Autodesk Fusion 360 part; units mm, degrees
(part 6 of 10)
sketch "Sketch33" plane through (0, 0, 9) normal (0, 0, 1) x (-1, 0, 0)
  line L0 (-20, 20.68) -> (-20, 19.68)
  line L1 (-20, 19.68) -> (-21, 19.68)
  line L2 (-21, 19.68) -> (-21, 20.68)
  line L3 (-21, 20.68) -> (-20, 20.68)
  line L4 (-23, 20.68) -> (-23, 19.68)
  line L5 (-23, 19.68) -> (-24, 19.68)
  line L6 (-24, 19.68) -> (-24, 20.68)
  line L7 (-24, 20.68) -> (-23, 20.68)
  line L8 (-20, 18.05) -> (-20, 17.05)
  line L9 (-20, 17.05) -> (-21, 17.05)
  line L10 (-21, 17.05) -> (-21, 18.05)
  line L11 (-21, 18.05) -> (-20, 18.05)
  line L12 (-23, 18.05) -> (-23, 17.05)
  line L13 (-23, 17.05) -> (-24, 17.05)
  line L14 (-24, 17.05) -> (-24, 18.05)
  line L15 (-24, 18.05) -> (-23, 18.05)
  line L16 (-20, 15.42) -> (-20, 14.42)
  line L17 (-20, 14.42) -> (-21, 14.42)
  line L18 (-21, 14.42) -> (-21, 15.42)
  line L19 (-21, 15.42) -> (-20, 15.42)
  line L20 (-23, 15.42) -> (-23, 14.42)
  line L21 (-23, 14.42) -> (-24, 14.42)
  line L22 (-24, 14.42) -> (-24, 15.42)
  line L23 (-24, 15.42) -> (-23, 15.42)
  line L24 (-20, 12.79) -> (-20, 11.79)
  line L25 (-20, 11.79) -> (-21, 11.79)
  line L26 (-21, 11.79) -> (-21, 12.79)
  line L27 (-21, 12.79) -> (-20, 12.79)
  line L28 (-23, 12.79) -> (-23, 11.79)
  line L29 (-23, 11.79) -> (-24, 11.79)
  line L30 (-24, 11.79) -> (-24, 12.79)
  line L31 (-24, 12.79) -> (-23, 12.79)
  line L32 (-20, 10.16) -> (-20, 9.16)
  line L33 (-20, 9.16) -> (-21, 9.16)
  line L34 (-21, 9.16) -> (-21, 10.16)
  line L35 (-21, 10.16) -> (-20, 10.16)
  line L36 (-23, 10.16) -> (-23, 9.16)
  line L37 (-23, 9.16) -> (-24, 9.16)
  line L38 (-24, 9.16) -> (-24, 10.16)
  line L39 (-24, 10.16) -> (-23, 10.16)
  line L40 (-19.998, 5.46) -> (-19.998, 4.46)
  line L41 (-19.998, 4.46) -> (-20.998, 4.46)
  line L42 (-20.998, 4.46) -> (-20.998, 5.46)
  line L43 (-20.998, 5.46) -> (-19.998, 5.46)
  line L44 (-22.998, 5.46) -> (-22.998, 4.46)
  line L45 (-22.998, 4.46) -> (-23.998, 4.46)
  line L46 (-23.998, 4.46) -> (-23.998, 5.46)
  line L47 (-23.998, 5.46) -> (-22.998, 5.46)
  line L48 (-19.998, 2.83) -> (-19.998, 1.83)
  line L49 (-19.998, 1.83) -> (-20.998, 1.83)
  line L50 (-20.998, 1.83) -> (-20.998, 2.83)
  line L51 (-20.998, 2.83) -> (-19.998, 2.83)
  line L52 (-22.998, 2.83) -> (-22.998, 1.83)
  line L53 (-22.998, 1.83) -> (-23.998, 1.83)
  line L54 (-23.998, 1.83) -> (-23.998, 2.83)
  line L55 (-23.998, 2.83) -> (-22.998, 2.83)
  line L56 (-19.998, 0.2) -> (-19.998, -0.8)
  line L57 (-19.998, -0.8) -> (-20.998, -0.8)
  line L58 (-20.998, -0.8) -> (-20.998, 0.2)
  line L59 (-20.998, 0.2) -> (-19.998, 0.2)
  line L60 (-22.998, 0.2) -> (-22.998, -0.8)
  line L61 (-22.998, -0.8) -> (-23.998, -0.8)
  line L62 (-23.998, -0.8) -> (-23.998, 0.2)
  line L63 (-23.998, 0.2) -> (-22.998, 0.2)
  line L64 (-19.998, -2.43) -> (-19.998, -3.43)
  line L65 (-19.998, -3.43) -> (-20.998, -3.43)
  line L66 (-20.998, -3.43) -> (-20.998, -2.43)
  line L67 (-20.998, -2.43) -> (-19.998, -2.43)
  line L68 (-22.998, -2.43) -> (-22.998, -3.43)
  line L69 (-22.998, -3.43) -> (-23.998, -3.43)
  line L70 (-23.998, -3.43) -> (-23.998, -2.43)
  line L71 (-23.998, -2.43) -> (-22.998, -2.43)
  line L72 (-19.998, -5.06) -> (-19.998, -6.06)
  line L73 (-19.998, -6.06) -> (-20.998, -6.06)
  line L74 (-20.998, -6.06) -> (-20.998, -5.06)
  line L75 (-20.998, -5.06) -> (-19.998, -5.06)
  line L76 (-22.998, -5.06) -> (-22.998, -6.06)
  line L77 (-22.998, -6.06) -> (-23.998, -6.06)
  line L78 (-23.998, -6.06) -> (-23.998, -5.06)
  line L79 (-23.998, -5.06) -> (-22.998, -5.06)
  line L80 (-20, -9.76) -> (-20, -10.76)
  line L81 (-20, -10.76) -> (-21, -10.76)
  line L82 (-21, -10.76) -> (-21, -9.76)
  line L83 (-21, -9.76) -> (-20, -9.76)
  line L84 (-23, -9.76) -> (-23, -10.76)
  line L85 (-23, -10.76) -> (-24, -10.76)
  line L86 (-24, -10.76) -> (-24, -9.76)
  line L87 (-24, -9.76) -> (-23, -9.76)
  line L88 (-20, -12.39) -> (-20, -13.39)
  line L89 (-20, -13.39) -> (-21, -13.39)
  line L90 (-21, -13.39) -> (-21, -12.39)
  line L91 (-21, -12.39) -> (-20, -12.39)
  line L92 (-23, -12.39) -> (-23, -13.39)
  line L93 (-23, -13.39) -> (-24, -13.39)
  line L94 (-24, -13.39) -> (-24, -12.39)
  line L95 (-24, -12.39) -> (-23, -12.39)
  line L96 (-20, -15.02) -> (-20, -16.02)
  line L97 (-20, -16.02) -> (-21, -16.02)
  line L98 (-21, -16.02) -> (-21, -15.02)
  line L99 (-21, -15.02) -> (-20, -15.02)
  line L100 (-23, -15.02) -> (-23, -16.02)
  line L101 (-23, -16.02) -> (-24, -16.02)
  line L102 (-24, -16.02) -> (-24, -15.02)
  line L103 (-24, -15.02) -> (-23, -15.02)
  line L104 (-20, -17.65) -> (-20, -18.65)
  line L105 (-20, -18.65) -> (-21, -18.65)
  line L106 (-21, -18.65) -> (-21, -17.65)
  line L107 (-21, -17.65) -> (-20, -17.65)
  line L108 (-23, -17.65) -> (-23, -18.65)
  line L109 (-23, -18.65) -> (-24, -18.65)
  line L110 (-24, -18.65) -> (-24, -17.65)
  line L111 (-24, -17.65) -> (-23, -17.65)
  line L112 (-20, -20.28) -> (-20, -21.28)
  line L113 (-20, -21.28) -> (-21, -21.28)
  line L114 (-21, -21.28) -> (-21, -20.28)
  line L115 (-21, -20.28) -> (-20, -20.28)
  line L116 (-23, -20.28) -> (-23, -21.28)
  line L117 (-23, -21.28) -> (-24, -21.28)
  line L118 (-24, -21.28) -> (-24, -20.28)
  line L119 (-24, -20.28) -> (-23, -20.28)
  line L120 (-20, -24.98) -> (-20, -25.98)
  line L121 (-20, -25.98) -> (-21, -25.98)
  line L122 (-21, -25.98) -> (-21, -24.98)
  line L123 (-21, -24.98) -> (-20, -24.98)
  line L124 (-23, -24.98) -> (-23, -25.98)
  line L125 (-23, -25.98) -> (-24, -25.98)
  line L126 (-24, -25.98) -> (-24, -24.98)
  line L127 (-24, -24.98) -> (-23, -24.98)
  line L128 (-20, -27.61) -> (-20, -28.61)
  line L129 (-20, -28.61) -> (-21, -28.61)
  line L130 (-21, -28.61) -> (-21, -27.61)
  line L131 (-21, -27.61) -> (-20, -27.61)
  line L132 (-23, -27.61) -> (-23, -28.61)
  line L133 (-23, -28.61) -> (-24, -28.61)
  line L134 (-24, -28.61) -> (-24, -27.61)
  line L135 (-24, -27.61) -> (-23, -27.61)
  line L136 (-20, -30.24) -> (-20, -31.24)
  line L137 (-20, -31.24) -> (-21, -31.24)
  line L138 (-21, -31.24) -> (-21, -30.24)
  line L139 (-21, -30.24) -> (-20, -30.24)
  line L140 (-23, -30.24) -> (-23, -31.24)
  line L141 (-23, -31.24) -> (-24, -31.24)
  line L142 (-24, -31.24) -> (-24, -30.24)
  line L143 (-24, -30.24) -> (-23, -30.24)
  line L144 (-20, -32.87) -> (-20, -33.87)
  line L145 (-20, -33.87) -> (-21, -33.87)
  line L146 (-21, -33.87) -> (-21, -32.87)
  line L147 (-21, -32.87) -> (-20, -32.87)
  line L148 (-23, -32.87) -> (-23, -33.87)
  line L149 (-23, -33.87) -> (-24, -33.87)
  line L150 (-24, -33.87) -> (-24, -32.87)
  line L151 (-24, -32.87) -> (-23, -32.87)
  line L152 (-20, -35.5) -> (-20, -36.5)
  line L153 (-20, -36.5) -> (-21, -36.5)
  line L154 (-21, -36.5) -> (-21, -35.5)
  line L155 (-21, -35.5) -> (-20, -35.5)
  line L156 (-23, -35.5) -> (-23, -36.5)
  line L157 (-23, -36.5) -> (-24, -36.5)
  line L158 (-24, -36.5) -> (-24, -35.5)
  line L159 (-24, -35.5) -> (-23, -35.5)
  line L160 (-13.7, 38.77) -> (-13.7, 37.77)
  line L161 (-13.7, 37.77) -> (-14.7, 37.77)
  line L162 (-14.7, 37.77) -> (-14.7, 38.77)
  line L163 (-14.7, 38.77) -> (-13.7, 38.77)
  line L164 (-13.7, 36.14) -> (-13.7, 35.14)
  line L165 (-13.7, 35.14) -> (-14.7, 35.14)
  line L166 (-14.7, 35.14) -> (-14.7, 36.14)
  line L167 (-14.7, 36.14) -> (-13.7, 36.14)
  line L168 (-13.7, 33.51) -> (-13.7, 32.51)
  line L169 (-13.7, 32.51) -> (-14.7, 32.51)
  line L170 (-14.7, 32.51) -> (-14.7, 33.51)
  line L171 (-14.7, 33.51) -> (-13.7, 33.51)
  line L172 (-13.7, 30.88) -> (-13.7, 29.88)
  line L173 (-13.7, 29.88) -> (-14.7, 29.88)
  line L174 (-14.7, 29.88) -> (-14.7, 30.88)
  line L175 (-14.7, 30.88) -> (-13.7, 30.88)
  line L176 (-13.7, 28.25) -> (-13.7, 27.25)
  line L177 (-13.7, 27.25) -> (-14.7, 27.25)
  line L178 (-14.7, 27.25) -> (-14.7, 28.25)
  line L179 (-14.7, 28.25) -> (-13.7, 28.25)
  line L180 (-13.7, 25.62) -> (-13.7, 24.62)
  line L181 (-13.7, 24.62) -> (-14.7, 24.62)
  line L182 (-14.7, 24.62) -> (-14.7, 25.62)
  line L183 (-14.7, 25.62) -> (-13.7, 25.62)
  line L184 (-13.7, 22.99) -> (-13.7, 21.99)
  line L185 (-13.7, 21.99) -> (-14.7, 21.99)
  line L186 (-14.7, 21.99) -> (-14.7, 22.99)
  line L187 (-14.7, 22.99) -> (-13.7, 22.99)
  line L188 (-13.7, 20.36) -> (-13.7, 19.36)
  line L189 (-13.7, 19.36) -> (-14.7, 19.36)
  line L190 (-14.7, 19.36) -> (-14.7, 20.36)
  line L191 (-14.7, 20.36) -> (-13.7, 20.36)
  line L192 (-13.7, 17.73) -> (-13.7, 16.73)
  line L193 (-13.7, 16.73) -> (-14.7, 16.73)
  line L194 (-14.7, 16.73) -> (-14.7, 17.73)
  line L195 (-14.7, 17.73) -> (-13.7, 17.73)
  line L196 (-13.7, 15.1) -> (-13.7, 14.1)
  line L197 (-13.7, 14.1) -> (-14.7, 14.1)
  line L198 (-14.7, 14.1) -> (-14.7, 15.1)
  line L199 (-14.7, 15.1) -> (-13.7, 15.1)
  line L200 (-13.7, 12.47) -> (-13.7, 11.47)
  line L201 (-13.7, 11.47) -> (-14.7, 11.47)
  line L202 (-14.7, 11.47) -> (-14.7, 12.47)
  line L203 (-14.7, 12.47) -> (-13.7, 12.47)
  line L204 (-13.7, 9.84) -> (-13.7, 8.84)
  line L205 (-13.7, 8.84) -> (-14.7, 8.84)
  line L206 (-14.7, 8.84) -> (-14.7, 9.84)
  line L207 (-14.7, 9.84) -> (-13.7, 9.84)
  line L208 (-13.7, 7.21) -> (-13.7, 6.21)
  line L209 (-13.7, 6.21) -> (-14.7, 6.21)
  line L210 (-14.7, 6.21) -> (-14.7, 7.21)
  line L211 (-14.7, 7.21) -> (-13.7, 7.21)
  line L212 (-13.7, 4.58) -> (-13.7, 3.58)
  line L213 (-13.7, 3.58) -> (-14.7, 3.58)
  line L214 (-14.7, 3.58) -> (-14.7, 4.58)
  line L215 (-14.7, 4.58) -> (-13.7, 4.58)
  line L216 (-13.7, 1.95) -> (-13.7, 0.95)
  line L217 (-13.7, 0.95) -> (-14.7, 0.95)
  line L218 (-14.7, 0.95) -> (-14.7, 1.95)
  line L219 (-14.7, 1.95) -> (-13.7, 1.95)
  line L220 (-13.7, -0.68) -> (-13.7, -1.68)
  line L221 (-13.7, -1.68) -> (-14.7, -1.68)
  line L222 (-14.7, -1.68) -> (-14.7, -0.68)
  line L223 (-14.7, -0.68) -> (-13.7, -0.68)
  line L224 (-13.7, -3.31) -> (-13.7, -4.31)
  line L225 (-13.7, -4.31) -> (-14.7, -4.31)
  line L226 (-14.7, -4.31) -> (-14.7, -3.31)
  line L227 (-14.7, -3.31) -> (-13.7, -3.31)
  line L228 (-13.7, -5.94) -> (-13.7, -6.94)
  line L229 (-13.7, -6.94) -> (-14.7, -6.94)
  line L230 (-14.7, -6.94) -> (-14.7, -5.94)
  line L231 (-14.7, -5.94) -> (-13.7, -5.94)
  line L232 (-13.7, -8.57) -> (-13.7, -9.57)
  line L233 (-13.7, -9.57) -> (-14.7, -9.57)
  line L234 (-14.7, -9.57) -> (-14.7, -8.57)
  line L235 (-14.7, -8.57) -> (-13.7, -8.57)
  line L236 (-13.7, -11.2) -> (-13.7, -12.2)
  line L237 (-13.7, -12.2) -> (-14.7, -12.2)
  line L238 (-14.7, -12.2) -> (-14.7, -11.2)
  line L239 (-14.7, -11.2) -> (-13.7, -11.2)
  line L240 (-13.7, -13.83) -> (-13.7, -14.83)
  line L241 (-13.7, -14.83) -> (-14.7, -14.83)
  line L242 (-14.7, -14.83) -> (-14.7, -13.83)
  line L243 (-14.7, -13.83) -> (-13.7, -13.83)
  line L244 (-13.7, -16.46) -> (-13.7, -17.46)
  line L245 (-13.7, -17.46) -> (-14.7, -17.46)
  line L246 (-14.7, -17.46) -> (-14.7, -16.46)
  line L247 (-14.7, -16.46) -> (-13.7, -16.46)
  line L248 (-13.7, -19.09) -> (-13.7, -20.09)
  line L249 (-13.7, -20.09) -> (-14.7, -20.09)
  line L250 (-14.7, -20.09) -> (-14.7, -19.09)
  line L251 (-14.7, -19.09) -> (-13.7, -19.09)
  line L252 (-13.7, -21.72) -> (-13.7, -22.72)
  line L253 (-13.7, -22.72) -> (-14.7, -22.72)
  line L254 (-14.7, -22.72) -> (-14.7, -21.72)
  line L255 (-14.7, -21.72) -> (-13.7, -21.72)
  line L256 (-13.7, -24.35) -> (-13.7, -25.35)
  line L257 (-13.7, -25.35) -> (-14.7, -25.35)
  line L258 (-14.7, -25.35) -> (-14.7, -24.35)
  line L259 (-14.7, -24.35) -> (-13.7, -24.35)
  line L260 (-13.7, -26.98) -> (-13.7, -27.98)
  line L261 (-13.7, -27.98) -> (-14.7, -27.98)
  line L262 (-14.7, -27.98) -> (-14.7, -26.98)
  line L263 (-14.7, -26.98) -> (-13.7, -26.98)
  line L264 (-13.7, -29.61) -> (-13.7, -30.61)
  line L265 (-13.7, -30.61) -> (-14.7, -30.61)
  line L266 (-14.7, -30.61) -> (-14.7, -29.61)
  line L267 (-14.7, -29.61) -> (-13.7, -29.61)
  line L268 (-13.7, -32.24) -> (-13.7, -33.24)
  line L269 (-13.7, -33.24) -> (-14.7, -33.24)
  line L270 (-14.7, -33.24) -> (-14.7, -32.24)
  line L271 (-14.7, -32.24) -> (-13.7, -32.24)
  line L272 (-13.7, -34.87) -> (-13.7, -35.87)
  line L273 (-13.7, -35.87) -> (-14.7, -35.87)
  line L274 (-14.7, -35.87) -> (-14.7, -34.87)
  line L275 (-14.7, -34.87) -> (-13.7, -34.87)
  line L276 (-13.7, -37.5) -> (-13.7, -38.5)
  line L277 (-13.7, -38.5) -> (-14.7, -38.5)
  line L278 (-14.7, -38.5) -> (-14.7, -37.5)
  line L279 (-14.7, -37.5) -> (-13.7, -37.5)
  line L280 (-10.9, 38.77) -> (-10.9, 37.77)
  line L281 (-10.9, 37.77) -> (-11.9, 37.77)
  line L282 (-11.9, 37.77) -> (-11.9, 38.77)
  line L283 (-11.9, 38.77) -> (-10.9, 38.77)
  line L284 (-10.9, 36.14) -> (-10.9, 35.14)
  line L285 (-10.9, 35.14) -> (-11.9, 35.14)
  line L286 (-11.9, 35.14) -> (-11.9, 36.14)
  line L287 (-11.9, 36.14) -> (-10.9, 36.14)
  line L288 (-10.9, 33.51) -> (-10.9, 32.51)
  line L289 (-10.9, 32.51) -> (-11.9, 32.51)
  line L290 (-11.9, 32.51) -> (-11.9, 33.51)
  line L291 (-11.9, 33.51) -> (-10.9, 33.51)
  line L292 (-10.9, 30.88) -> (-10.9, 29.88)
  line L293 (-10.9, 29.88) -> (-11.9, 29.88)
  line L294 (-11.9, 29.88) -> (-11.9, 30.88)
  line L295 (-11.9, 30.88) -> (-10.9, 30.88)
  line L296 (-10.9, 28.25) -> (-10.9, 27.25)
  line L297 (-10.9, 27.25) -> (-11.9, 27.25)
  line L298 (-11.9, 27.25) -> (-11.9, 28.25)
  line L299 (-11.9, 28.25) -> (-10.9, 28.25)
  line L300 (-10.9, 25.62) -> (-10.9, 24.62)
  line L301 (-10.9, 24.62) -> (-11.9, 24.62)
  line L302 (-11.9, 24.62) -> (-11.9, 25.62)
  line L303 (-11.9, 25.62) -> (-10.9, 25.62)
  line L304 (-10.9, 22.99) -> (-10.9, 21.99)
  line L305 (-10.9, 21.99) -> (-11.9, 21.99)
  line L306 (-11.9, 21.99) -> (-11.9, 22.99)
  line L307 (-11.9, 22.99) -> (-10.9, 22.99)
  line L308 (-10.9, 20.36) -> (-10.9, 19.36)
  line L309 (-10.9, 19.36) -> (-11.9, 19.36)
  line L310 (-11.9, 19.36) -> (-11.9, 20.36)
  line L311 (-11.9, 20.36) -> (-10.9, 20.36)
  line L312 (-10.9, 17.73) -> (-10.9, 16.73)
  line L313 (-10.9, 16.73) -> (-11.9, 16.73)
  line L314 (-11.9, 16.73) -> (-11.9, 17.73)
  line L315 (-11.9, 17.73) -> (-10.9, 17.73)
  line L316 (-10.9, 15.1) -> (-10.9, 14.1)
  line L317 (-10.9, 14.1) -> (-11.9, 14.1)
  line L318 (-11.9, 14.1) -> (-11.9, 15.1)
  line L319 (-11.9, 15.1) -> (-10.9, 15.1)
  line L320 (-10.9, 12.47) -> (-10.9, 11.47)
  line L321 (-10.9, 11.47) -> (-11.9, 11.47)
  line L322 (-11.9, 11.47) -> (-11.9, 12.47)
  line L323 (-11.9, 12.47) -> (-10.9, 12.47)
  line L324 (-10.9, 9.84) -> (-10.9, 8.84)
  line L325 (-10.9, 8.84) -> (-11.9, 8.84)
  line L326 (-11.9, 8.84) -> (-11.9, 9.84)
  line L327 (-11.9, 9.84) -> (-10.9, 9.84)
  line L328 (-10.9, 7.21) -> (-10.9, 6.21)
  line L329 (-10.9, 6.21) -> (-11.9, 6.21)
  line L330 (-11.9, 6.21) -> (-11.9, 7.21)
  line L331 (-11.9, 7.21) -> (-10.9, 7.21)
  line L332 (-10.9, 4.58) -> (-10.9, 3.58)
  line L333 (-10.9, 3.58) -> (-11.9, 3.58)
  line L334 (-11.9, 3.58) -> (-11.9, 4.58)
  line L335 (-11.9, 4.58) -> (-10.9, 4.58)
  line L336 (-10.9, 1.95) -> (-10.9, 0.95)
  line L337 (-10.9, 0.95) -> (-11.9, 0.95)
  line L338 (-11.9, 0.95) -> (-11.9, 1.95)
  line L339 (-11.9, 1.95) -> (-10.9, 1.95)
  line L340 (-10.9, -0.68) -> (-10.9, -1.68)
  line L341 (-10.9, -1.68) -> (-11.9, -1.68)
  line L342 (-11.9, -1.68) -> (-11.9, -0.68)
  line L343 (-11.9, -0.68) -> (-10.9, -0.68)
  line L344 (-10.9, -3.31) -> (-10.9, -4.31)
  line L345 (-10.9, -4.31) -> (-11.9, -4.31)
  line L346 (-11.9, -4.31) -> (-11.9, -3.31)
  line L347 (-11.9, -3.31) -> (-10.9, -3.31)
  line L348 (-10.9, -5.94) -> (-10.9, -6.94)
  line L349 (-10.9, -6.94) -> (-11.9, -6.94)
  line L350 (-11.9, -6.94) -> (-11.9, -5.94)
  line L351 (-11.9, -5.94) -> (-10.9, -5.94)
  line L352 (-10.9, -8.57) -> (-10.9, -9.57)
  line L353 (-10.9, -9.57) -> (-11.9, -9.57)
  line L354 (-11.9, -9.57) -> (-11.9, -8.57)
  line L355 (-11.9, -8.57) -> (-10.9, -8.57)
  line L356 (-10.9, -11.2) -> (-10.9, -12.2)
  line L357 (-10.9, -12.2) -> (-11.9, -12.2)
  line L358 (-11.9, -12.2) -> (-11.9, -11.2)
  line L359 (-11.9, -11.2) -> (-10.9, -11.2)
  line L360 (-10.9, -13.83) -> (-10.9, -14.83)
  line L361 (-10.9, -14.83) -> (-11.9, -14.83)
  line L362 (-11.9, -14.83) -> (-11.9, -13.83)
  line L363 (-11.9, -13.83) -> (-10.9, -13.83)
  line L364 (-10.9, -16.46) -> (-10.9, -17.46)
  line L365 (-10.9, -17.46) -> (-11.9, -17.46)
  line L366 (-11.9, -17.46) -> (-11.9, -16.46)
  line L367 (-11.9, -16.46) -> (-10.9, -16.46)
  line L368 (-10.9, -19.09) -> (-10.9, -20.09)
  line L369 (-10.9, -20.09) -> (-11.9, -20.09)
  line L370 (-11.9, -20.09) -> (-11.9, -19.09)
  line L371 (-11.9, -19.09) -> (-10.9, -19.09)
  line L372 (-10.9, -21.72) -> (-10.9, -22.72)
  line L373 (-10.9, -22.72) -> (-11.9, -22.72)
  line L374 (-11.9, -22.72) -> (-11.9, -21.72)
  line L375 (-11.9, -21.72) -> (-10.9, -21.72)
  line L376 (-10.9, -24.35) -> (-10.9, -25.35)
  line L377 (-10.9, -25.35) -> (-11.9, -25.35)
  line L378 (-11.9, -25.35) -> (-11.9, -24.35)
  line L379 (-11.9, -24.35) -> (-10.9, -24.35)
  line L380 (-10.9, -26.98) -> (-10.9, -27.98)
  line L381 (-10.9, -27.98) -> (-11.9, -27.98)
  line L382 (-11.9, -27.98) -> (-11.9, -26.98)
  line L383 (-11.9, -26.98) -> (-10.9, -26.98)
  line L384 (-10.9, -29.61) -> (-10.9, -30.61)
  line L385 (-10.9, -30.61) -> (-11.9, -30.61)
  line L386 (-11.9, -30.61) -> (-11.9, -29.61)
  line L387 (-11.9, -29.61) -> (-10.9, -29.61)
  line L388 (-10.9, -32.24) -> (-10.9, -33.24)
  line L389 (-10.9, -33.24) -> (-11.9, -33.24)
  line L390 (-11.9, -33.24) -> (-11.9, -32.24)
  line L391 (-11.9, -32.24) -> (-10.9, -32.24)
  line L392 (-10.9, -34.87) -> (-10.9, -35.87)
  line L393 (-10.9, -35.87) -> (-11.9, -35.87)
  line L394 (-11.9, -35.87) -> (-11.9, -34.87)
  line L395 (-11.9, -34.87) -> (-10.9, -34.87)
  line L396 (-10.9, -37.5) -> (-10.9, -38.5)
  line L397 (-10.9, -38.5) -> (-11.9, -38.5)
  line L398 (-11.9, -38.5) -> (-11.9, -37.5)
  line L399 (-11.9, -37.5) -> (-10.9, -37.5)
  line L400 (-8.1, 38.77) -> (-8.1, 37.77)
  line L401 (-8.1, 37.77) -> (-9.1, 37.77)
  line L402 (-9.1, 37.77) -> (-9.1, 38.77)
  line L403 (-9.1, 38.77) -> (-8.1, 38.77)
  line L404 (-8.1, 36.14) -> (-8.1, 35.14)
  line L405 (-8.1, 35.14) -> (-9.1, 35.14)
  line L406 (-9.1, 35.14) -> (-9.1, 36.14)
  line L407 (-9.1, 36.14) -> (-8.1, 36.14)
  line L408 (-8.1, 33.51) -> (-8.1, 32.51)
  line L409 (-8.1, 32.51) -> (-9.1, 32.51)
  line L410 (-9.1, 32.51) -> (-9.1, 33.51)
  line L411 (-9.1, 33.51) -> (-8.1, 33.51)
  line L412 (-8.1, 30.88) -> (-8.1, 29.88)
  line L413 (-8.1, 29.88) -> (-9.1, 29.88)
  line L414 (-9.1, 29.88) -> (-9.1, 30.88)
  line L415 (-9.1, 30.88) -> (-8.1, 30.88)
  line L416 (-8.1, 28.25) -> (-8.1, 27.25)
  line L417 (-8.1, 27.25) -> (-9.1, 27.25)
  line L418 (-9.1, 27.25) -> (-9.1, 28.25)
  line L419 (-9.1, 28.25) -> (-8.1, 28.25)
  line L420 (-8.1, 25.62) -> (-8.1, 24.62)
  line L421 (-8.1, 24.62) -> (-9.1, 24.62)
  line L422 (-9.1, 24.62) -> (-9.1, 25.62)
  line L423 (-9.1, 25.62) -> (-8.1, 25.62)
  line L424 (-8.1, 22.99) -> (-8.1, 21.99)
  line L425 (-8.1, 21.99) -> (-9.1, 21.99)
  line L426 (-9.1, 21.99) -> (-9.1, 22.99)
  line L427 (-9.1, 22.99) -> (-8.1, 22.99)
  line L428 (-8.1, 20.36) -> (-8.1, 19.36)
  line L429 (-8.1, 19.36) -> (-9.1, 19.36)
  line L430 (-9.1, 19.36) -> (-9.1, 20.36)
  line L431 (-9.1, 20.36) -> (-8.1, 20.36)
  line L432 (-8.1, 17.73) -> (-8.1, 16.73)
  line L433 (-8.1, 16.73) -> (-9.1, 16.73)
  line L434 (-9.1, 16.73) -> (-9.1, 17.73)
  line L435 (-9.1, 17.73) -> (-8.1, 17.73)
  line L436 (-8.1, 15.1) -> (-8.1, 14.1)
  line L437 (-8.1, 14.1) -> (-9.1, 14.1)
  line L438 (-9.1, 14.1) -> (-9.1, 15.1)
  line L439 (-9.1, 15.1) -> (-8.1, 15.1)
  line L440 (-8.1, 12.47) -> (-8.1, 11.47)
  line L441 (-8.1, 11.47) -> (-9.1, 11.47)
  line L442 (-9.1, 11.47) -> (-9.1, 12.47)
  line L443 (-9.1, 12.47) -> (-8.1, 12.47)
  line L444 (-8.1, 9.84) -> (-8.1, 8.84)
  line L445 (-8.1, 8.84) -> (-9.1, 8.84)
  line L446 (-9.1, 8.84) -> (-9.1, 9.84)
  line L447 (-9.1, 9.84) -> (-8.1, 9.84)
  line L448 (-8.1, 7.21) -> (-8.1, 6.21)
  line L449 (-8.1, 6.21) -> (-9.1, 6.21)
  line L450 (-9.1, 6.21) -> (-9.1, 7.21)
  line L451 (-9.1, 7.21) -> (-8.1, 7.21)
  line L452 (-8.1, 4.58) -> (-8.1, 3.58)
  line L453 (-8.1, 3.58) -> (-9.1, 3.58)
  line L454 (-9.1, 3.58) -> (-9.1, 4.58)
  line L455 (-9.1, 4.58) -> (-8.1, 4.58)
  line L456 (-8.1, 1.95) -> (-8.1, 0.95)
  line L457 (-8.1, 0.95) -> (-9.1, 0.95)
  line L458 (-9.1, 0.95) -> (-9.1, 1.95)
  line L459 (-9.1, 1.95) -> (-8.1, 1.95)
  line L460 (-8.1, -0.68) -> (-8.1, -1.68)
  line L461 (-8.1, -1.68) -> (-9.1, -1.68)
  line L462 (-9.1, -1.68) -> (-9.1, -0.68)
  line L463 (-9.1, -0.68) -> (-8.1, -0.68)
  line L464 (-8.1, -3.31) -> (-8.1, -4.31)
  line L465 (-8.1, -4.31) -> (-9.1, -4.31)
  line L466 (-9.1, -4.31) -> (-9.1, -3.31)
  line L467 (-9.1, -3.31) -> (-8.1, -3.31)
  line L468 (-8.1, -5.94) -> (-8.1, -6.94)
  line L469 (-8.1, -6.94) -> (-9.1, -6.94)
  line L470 (-9.1, -6.94) -> (-9.1, -5.94)
  line L471 (-9.1, -5.94) -> (-8.1, -5.94)
  line L472 (-8.1, -8.57) -> (-8.1, -9.57)
  line L473 (-8.1, -9.57) -> (-9.1, -9.57)
  line L474 (-9.1, -9.57) -> (-9.1, -8.57)
  line L475 (-9.1, -8.57) -> (-8.1, -8.57)
  line L476 (-8.1, -11.2) -> (-8.1, -12.2)
  line L477 (-8.1, -12.2) -> (-9.1, -12.2)
  line L478 (-9.1, -12.2) -> (-9.1, -11.2)
  line L479 (-9.1, -11.2) -> (-8.1, -11.2)
  line L480 (-8.1, -13.83) -> (-8.1, -14.83)
  line L481 (-8.1, -14.83) -> (-9.1, -14.83)
  line L482 (-9.1, -14.83) -> (-9.1, -13.83)
  line L483 (-9.1, -13.83) -> (-8.1, -13.83)
  line L484 (-8.1, -16.46) -> (-8.1, -17.46)
  line L485 (-8.1, -17.46) -> (-9.1, -17.46)
  line L486 (-9.1, -17.46) -> (-9.1, -16.46)
  line L487 (-9.1, -16.46) -> (-8.1, -16.46)
  line L488 (-8.1, -19.09) -> (-8.1, -20.09)
  line L489 (-8.1, -20.09) -> (-9.1, -20.09)
  line L490 (-9.1, -20.09) -> (-9.1, -19.09)
  line L491 (-9.1, -19.09) -> (-8.1, -19.09)
  line L492 (-8.1, -21.72) -> (-8.1, -22.72)
  line L493 (-8.1, -22.72) -> (-9.1, -22.72)
  line L494 (-9.1, -22.72) -> (-9.1, -21.72)
  line L495 (-9.1, -21.72) -> (-8.1, -21.72)
  line L496 (-8.1, -24.35) -> (-8.1, -25.35)
  line L497 (-8.1, -25.35) -> (-9.1, -25.35)
  line L498 (-9.1, -25.35) -> (-9.1, -24.35)
  line L499 (-9.1, -24.35) -> (-8.1, -24.35)
  line L500 (-8.1, -26.98) -> (-8.1, -27.98)
  line L501 (-8.1, -27.98) -> (-9.1, -27.98)
  line L502 (-9.1, -27.98) -> (-9.1, -26.98)
  line L503 (-9.1, -26.98) -> (-8.1, -26.98)
  line L504 (-8.1, -29.61) -> (-8.1, -30.61)
  line L505 (-8.1, -30.61) -> (-9.1, -30.61)
  line L506 (-9.1, -30.61) -> (-9.1, -29.61)
  line L507 (-9.1, -29.61) -> (-8.1, -29.61)
  line L508 (-8.1, -32.24) -> (-8.1, -33.24)
  line L509 (-8.1, -33.24) -> (-9.1, -33.24)
  line L510 (-9.1, -33.24) -> (-9.1, -32.24)
  line L511 (-9.1, -32.24) -> (-8.1, -32.24)
  line L512 (-8.1, -34.87) -> (-8.1, -35.87)
  line L513 (-8.1, -35.87) -> (-9.1, -35.87)
  line L514 (-9.1, -35.87) -> (-9.1, -34.87)
  line L515 (-9.1, -34.87) -> (-8.1, -34.87)
  line L516 (-8.1, -37.5) -> (-8.1, -38.5)
  line L517 (-8.1, -38.5) -> (-9.1, -38.5)
  line L518 (-9.1, -38.5) -> (-9.1, -37.5)
  line L519 (-9.1, -37.5) -> (-8.1, -37.5)
  line L520 (-5.3, 38.77) -> (-5.3, 37.77)
  line L521 (-5.3, 37.77) -> (-6.3, 37.77)
  line L522 (-6.3, 37.77) -> (-6.3, 38.77)
  line L523 (-6.3, 38.77) -> (-5.3, 38.77)
  line L524 (-5.3, 36.14) -> (-5.3, 35.14)
  line L525 (-5.3, 35.14) -> (-6.3, 35.14)
  line L526 (-6.3, 35.14) -> (-6.3, 36.14)
  line L527 (-6.3, 36.14) -> (-5.3, 36.14)
  line L528 (-5.3, 33.51) -> (-5.3, 32.51)
  line L529 (-5.3, 32.51) -> (-6.3, 32.51)
  line L530 (-6.3, 32.51) -> (-6.3, 33.51)
  line L531 (-6.3, 33.51) -> (-5.3, 33.51)
  line L532 (-5.3, 30.88) -> (-5.3, 29.88)
  line L533 (-5.3, 29.88) -> (-6.3, 29.88)
  line L534 (-6.3, 29.88) -> (-6.3, 30.88)
  line L535 (-6.3, 30.88) -> (-5.3, 30.88)
  line L536 (-5.3, 28.25) -> (-5.3, 27.25)
  line L537 (-5.3, 27.25) -> (-6.3, 27.25)
  line L538 (-6.3, 27.25) -> (-6.3, 28.25)
  line L539 (-6.3, 28.25) -> (-5.3, 28.25)
  line L540 (-5.3, 25.62) -> (-5.3, 24.62)
  line L541 (-5.3, 24.62) -> (-6.3, 24.62)
  line L542 (-6.3, 24.62) -> (-6.3, 25.62)
  line L543 (-6.3, 25.62) -> (-5.3, 25.62)
  line L544 (-5.3, 22.99) -> (-5.3, 21.99)
  line L545 (-5.3, 21.99) -> (-6.3, 21.99)
  line L546 (-6.3, 21.99) -> (-6.3, 22.99)
  line L547 (-6.3, 22.99) -> (-5.3, 22.99)
  line L548 (-5.3, 20.36) -> (-5.3, 19.36)
  line L549 (-5.3, 19.36) -> (-6.3, 19.36)
  line L550 (-6.3, 19.36) -> (-6.3, 20.36)
  line L551 (-6.3, 20.36) -> (-5.3, 20.36)
  line L552 (-5.3, 17.73) -> (-5.3, 16.73)
  line L553 (-5.3, 16.73) -> (-6.3, 16.73)
  line L554 (-6.3, 16.73) -> (-6.3, 17.73)
  line L555 (-6.3, 17.73) -> (-5.3, 17.73)
  line L556 (-5.3, 15.1) -> (-5.3, 14.1)
  line L557 (-5.3, 14.1) -> (-6.3, 14.1)
  line L558 (-6.3, 14.1) -> (-6.3, 15.1)
  line L559 (-6.3, 15.1) -> (-5.3, 15.1)
  line L560 (-5.3, 12.47) -> (-5.3, 11.47)
  line L561 (-5.3, 11.47) -> (-6.3, 11.47)
  line L562 (-6.3, 11.47) -> (-6.3, 12.47)
  line L563 (-6.3, 12.47) -> (-5.3, 12.47)
  line L564 (-5.3, 9.84) -> (-5.3, 8.84)
  line L565 (-5.3, 8.84) -> (-6.3, 8.84)
  line L566 (-6.3, 8.84) -> (-6.3, 9.84)
  line L567 (-6.3, 9.84) -> (-5.3, 9.84)
  line L568 (-5.3, 7.21) -> (-5.3, 6.21)
  line L569 (-5.3, 6.21) -> (-6.3, 6.21)
  line L570 (-6.3, 6.21) -> (-6.3, 7.21)
  line L571 (-6.3, 7.21) -> (-5.3, 7.21)
  line L572 (-5.3, 4.58) -> (-5.3, 3.58)
  line L573 (-5.3, 3.58) -> (-6.3, 3.58)
  line L574 (-6.3, 3.58) -> (-6.3, 4.58)
  line L575 (-6.3, 4.58) -> (-5.3, 4.58)
  line L576 (-5.3, 1.95) -> (-5.3, 0.95)
  line L577 (-5.3, 0.95) -> (-6.3, 0.95)
  line L578 (-6.3, 0.95) -> (-6.3, 1.95)
  line L579 (-6.3, 1.95) -> (-5.3, 1.95)
  line L580 (-5.3, -0.68) -> (-5.3, -1.68)
  line L581 (-5.3, -1.68) -> (-6.3, -1.68)
  line L582 (-6.3, -1.68) -> (-6.3, -0.68)
  line L583 (-6.3, -0.68) -> (-5.3, -0.68)
  line L584 (-5.3, -3.31) -> (-5.3, -4.31)
  line L585 (-5.3, -4.31) -> (-6.3, -4.31)
  line L586 (-6.3, -4.31) -> (-6.3, -3.31)
  line L587 (-6.3, -3.31) -> (-5.3, -3.31)
  line L588 (-5.3, -5.94) -> (-5.3, -6.94)
  line L589 (-5.3, -6.94) -> (-6.3, -6.94)
  line L590 (-6.3, -6.94) -> (-6.3, -5.94)
  line L591 (-6.3, -5.94) -> (-5.3, -5.94)
  line L592 (-5.3, -8.57) -> (-5.3, -9.57)
  line L593 (-5.3, -9.57) -> (-6.3, -9.57)
  line L594 (-6.3, -9.57) -> (-6.3, -8.57)
  line L595 (-6.3, -8.57) -> (-5.3, -8.57)
  line L596 (-5.3, -11.2) -> (-5.3, -12.2)
  line L597 (-5.3, -12.2) -> (-6.3, -12.2)
  line L598 (-6.3, -12.2) -> (-6.3, -11.2)
  line L599 (-6.3, -11.2) -> (-5.3, -11.2)
  line L600 (-5.3, -13.83) -> (-5.3, -14.83)
  line L601 (-5.3, -14.83) -> (-6.3, -14.83)
  line L602 (-6.3, -14.83) -> (-6.3, -13.83)
  line L603 (-6.3, -13.83) -> (-5.3, -13.83)
  line L604 (-5.3, -16.46) -> (-5.3, -17.46)
  line L605 (-5.3, -17.46) -> (-6.3, -17.46)
  line L606 (-6.3, -17.46) -> (-6.3, -16.46)
  line L607 (-6.3, -16.46) -> (-5.3, -16.46)
  line L608 (-5.3, -19.09) -> (-5.3, -20.09)
  line L609 (-5.3, -20.09) -> (-6.3, -20.09)
  line L610 (-6.3, -20.09) -> (-6.3, -19.09)
  line L611 (-6.3, -19.09) -> (-5.3, -19.09)
  line L612 (-5.3, -21.72) -> (-5.3, -22.72)
  line L613 (-5.3, -22.72) -> (-6.3, -22.72)
  line L614 (-6.3, -22.72) -> (-6.3, -21.72)
  line L615 (-6.3, -21.72) -> (-5.3, -21.72)
  line L616 (-5.3, -24.35) -> (-5.3, -25.35)
  line L617 (-5.3, -25.35) -> (-6.3, -25.35)
  line L618 (-6.3, -25.35) -> (-6.3, -24.35)
  line L619 (-6.3, -24.35) -> (-5.3, -24.35)
  line L620 (-5.3, -26.98) -> (-5.3, -27.98)
  line L621 (-5.3, -27.98) -> (-6.3, -27.98)
  line L622 (-6.3, -27.98) -> (-6.3, -26.98)
  line L623 (-6.3, -26.98) -> (-5.3, -26.98)
  line L624 (-5.3, -29.61) -> (-5.3, -30.61)
  line L625 (-5.3, -30.61) -> (-6.3, -30.61)
  line L626 (-6.3, -30.61) -> (-6.3, -29.61)
  line L627 (-6.3, -29.61) -> (-5.3, -29.61)
  line L628 (-5.3, -32.24) -> (-5.3, -33.24)
  line L629 (-5.3, -33.24) -> (-6.3, -33.24)
  line L630 (-6.3, -33.24) -> (-6.3, -32.24)
  line L631 (-6.3, -32.24) -> (-5.3, -32.24)
  line L632 (-5.3, -34.87) -> (-5.3, -35.87)
  line L633 (-5.3, -35.87) -> (-6.3, -35.87)
  line L634 (-6.3, -35.87) -> (-6.3, -34.87)
  line L635 (-6.3, -34.87) -> (-5.3, -34.87)
  line L636 (-5.3, -37.5) -> (-5.3, -38.5)
  line L637 (-5.3, -38.5) -> (-6.3, -38.5)
  line L638 (-6.3, -38.5) -> (-6.3, -37.5)
  line L639 (-6.3, -37.5) -> (-5.3, -37.5)
  line L640 (-2.5, 38.77) -> (-2.5, 37.77)
  line L641 (-2.5, 37.77) -> (-3.5, 37.77)
  line L642 (-3.5, 37.77) -> (-3.5, 38.77)
  line L643 (-3.5, 38.77) -> (-2.5, 38.77)
  line L644 (-2.5, 36.14) -> (-2.5, 35.14)
  line L645 (-2.5, 35.14) -> (-3.5, 35.14)
  line L646 (-3.5, 35.14) -> (-3.5, 36.14)
  line L647 (-3.5, 36.14) -> (-2.5, 36.14)
  line L648 (-2.5, 33.51) -> (-2.5, 32.51)
  line L649 (-2.5, 32.51) -> (-3.5, 32.51)
  line L650 (-3.5, 32.51) -> (-3.5, 33.51)
  line L651 (-3.5, 33.51) -> (-2.5, 33.51)
  line L652 (-2.5, 30.88) -> (-2.5, 29.88)
  line L653 (-2.5, 29.88) -> (-3.5, 29.88)
  line L654 (-3.5, 29.88) -> (-3.5, 30.88)
  line L655 (-3.5, 30.88) -> (-2.5, 30.88)
  line L656 (-2.5, 28.25) -> (-2.5, 27.25)
  line L657 (-2.5, 27.25) -> (-3.5, 27.25)
  line L658 (-3.5, 27.25) -> (-3.5, 28.25)
  line L659 (-3.5, 28.25) -> (-2.5, 28.25)
  line L660 (-2.5, 25.62) -> (-2.5, 24.62)
  line L661 (-2.5, 24.62) -> (-3.5, 24.62)
  line L662 (-3.5, 24.62) -> (-3.5, 25.62)
  line L663 (-3.5, 25.62) -> (-2.5, 25.62)
  line L664 (-2.5, 22.99) -> (-2.5, 21.99)
  line L665 (-2.5, 21.99) -> (-3.5, 21.99)
  line L666 (-3.5, 21.99) -> (-3.5, 22.99)
  line L667 (-3.5, 22.99) -> (-2.5, 22.99)
  line L668 (-2.5, 20.36) -> (-2.5, 19.36)
  line L669 (-2.5, 19.36) -> (-3.5, 19.36)
  line L670 (-3.5, 19.36) -> (-3.5, 20.36)
  line L671 (-3.5, 20.36) -> (-2.5, 20.36)
  line L672 (-2.5, 17.73) -> (-2.5, 16.73)
  line L673 (-2.5, 16.73) -> (-3.5, 16.73)
  line L674 (-3.5, 16.73) -> (-3.5, 17.73)
  line L675 (-3.5, 17.73) -> (-2.5, 17.73)
  line L676 (-2.5, 15.1) -> (-2.5, 14.1)
  line L677 (-2.5, 14.1) -> (-3.5, 14.1)
  line L678 (-3.5, 14.1) -> (-3.5, 15.1)
  line L679 (-3.5, 15.1) -> (-2.5, 15.1)
  line L680 (-2.5, 12.47) -> (-2.5, 11.47)
  line L681 (-2.5, 11.47) -> (-3.5, 11.47)
  line L682 (-3.5, 11.47) -> (-3.5, 12.47)
  line L683 (-3.5, 12.47) -> (-2.5, 12.47)
  line L684 (-2.5, 9.84) -> (-2.5, 8.84)
  line L685 (-2.5, 8.84) -> (-3.5, 8.84)
  line L686 (-3.5, 8.84) -> (-3.5, 9.84)
  line L687 (-3.5, 9.84) -> (-2.5, 9.84)
  line L688 (-2.5, 7.21) -> (-2.5, 6.21)
  line L689 (-2.5, 6.21) -> (-3.5, 6.21)
  line L690 (-3.5, 6.21) -> (-3.5, 7.21)
  line L691 (-3.5, 7.21) -> (-2.5, 7.21)
  line L692 (-2.5, 4.58) -> (-2.5, 3.58)
  line L693 (-2.5, 3.58) -> (-3.5, 3.58)
  line L694 (-3.5, 3.58) -> (-3.5, 4.58)
  line L695 (-3.5, 4.58) -> (-2.5, 4.58)
  line L696 (-2.5, 1.95) -> (-2.5, 0.95)
  line L697 (-2.5, 0.95) -> (-3.5, 0.95)
  line L698 (-3.5, 0.95) -> (-3.5, 1.95)
  line L699 (-3.5, 1.95) -> (-2.5, 1.95)
  line L700 (-2.5, -0.68) -> (-2.5, -1.68)
  line L701 (-2.5, -1.68) -> (-3.5, -1.68)
  line L702 (-3.5, -1.68) -> (-3.5, -0.68)
  line L703 (-3.5, -0.68) -> (-2.5, -0.68)
  line L704 (-2.5, -3.31) -> (-2.5, -4.31)
  line L705 (-2.5, -4.31) -> (-3.5, -4.31)
  line L706 (-3.5, -4.31) -> (-3.5, -3.31)
  line L707 (-3.5, -3.31) -> (-2.5, -3.31)
  line L708 (-2.5, -5.94) -> (-2.5, -6.94)
  line L709 (-2.5, -6.94) -> (-3.5, -6.94)
  line L710 (-3.5, -6.94) -> (-3.5, -5.94)
  line L711 (-3.5, -5.94) -> (-2.5, -5.94)
  line L712 (-2.5, -8.57) -> (-2.5, -9.57)
  line L713 (-2.5, -9.57) -> (-3.5, -9.57)
  line L714 (-3.5, -9.57) -> (-3.5, -8.57)
  line L715 (-3.5, -8.57) -> (-2.5, -8.57)
  line L716 (-2.5, -11.2) -> (-2.5, -12.2)
  line L717 (-2.5, -12.2) -> (-3.5, -12.2)
  line L718 (-3.5, -12.2) -> (-3.5, -11.2)
  line L719 (-3.5, -11.2) -> (-2.5, -11.2)
  line L720 (-2.5, -13.83) -> (-2.5, -14.83)
  line L721 (-2.5, -14.83) -> (-3.5, -14.83)
  line L722 (-3.5, -14.83) -> (-3.5, -13.83)
  line L723 (-3.5, -13.83) -> (-2.5, -13.83)
  line L724 (-2.5, -16.46) -> (-2.5, -17.46)
  line L725 (-2.5, -17.46) -> (-3.5, -17.46)
  line L726 (-3.5, -17.46) -> (-3.5, -16.46)
  line L727 (-3.5, -16.46) -> (-2.5, -16.46)
  line L728 (-2.5, -19.09) -> (-2.5, -20.09)
  line L729 (-2.5, -20.09) -> (-3.5, -20.09)
  line L730 (-3.5, -20.09) -> (-3.5, -19.09)
  line L731 (-3.5, -19.09) -> (-2.5, -19.09)
  line L732 (-2.5, -21.72) -> (-2.5, -22.72)
  line L733 (-2.5, -22.72) -> (-3.5, -22.72)
  line L734 (-3.5, -22.72) -> (-3.5, -21.72)
  line L735 (-3.5, -21.72) -> (-2.5, -21.72)
  line L736 (-2.5, -24.35) -> (-2.5, -25.35)
  line L737 (-2.5, -25.35) -> (-3.5, -25.35)
  line L738 (-3.5, -25.35) -> (-3.5, -24.35)
  line L739 (-3.5, -24.35) -> (-2.5, -24.35)
  line L740 (-2.5, -26.98) -> (-2.5, -27.98)
  line L741 (-2.5, -27.98) -> (-3.5, -27.98)
  line L742 (-3.5, -27.98) -> (-3.5, -26.98)
  line L743 (-3.5, -26.98) -> (-2.5, -26.98)
  line L744 (-2.5, -29.61) -> (-2.5, -30.61)
  line L745 (-2.5, -30.61) -> (-3.5, -30.61)
  line L746 (-3.5, -30.61) -> (-3.5, -29.61)
  line L747 (-3.5, -29.61) -> (-2.5, -29.61)
  line L748 (-2.5, -32.24) -> (-2.5, -33.24)
  line L749 (-2.5, -33.24) -> (-3.5, -33.24)
  line L750 (-3.5, -33.24) -> (-3.5, -32.24)
  line L751 (-3.5, -32.24) -> (-2.5, -32.24)
  line L752 (-2.5, -34.87) -> (-2.5, -35.87)
  line L753 (-2.5, -35.87) -> (-3.5, -35.87)
  line L754 (-3.5, -35.87) -> (-3.5, -34.87)
  line L755 (-3.5, -34.87) -> (-2.5, -34.87)
  line L756 (-2.5, -37.5) -> (-2.5, -38.5)
  line L757 (-2.5, -38.5) -> (-3.5, -38.5)
  line L758 (-3.5, -38.5) -> (-3.5, -37.5)
  line L759 (-3.5, -37.5) -> (-2.5, -37.5)
  line L760 (-1, -40.5) -> (-1, 40.5)
  line L761 (-1, 40.5) -> (-26.5, 40.5)
  line L762 (-26.5, 40.5) -> (-26.5, -40.5)
  line L763 (-26.5, -40.5) -> (-1, -40.5)
  line L764 (-24, 25.38) -> (-23, 25.38)
  line L765 (-23, 25.38) -> (-23, 24.38)
  line L766 (-23, 24.38) -> (-24, 24.38)
  line L767 (-24, 24.38) -> (-24, 25.38)
  line L768 (-24, 25.38) -> (-23, 24.38) construction
  line L769 (-23, 25.38) -> (-24, 24.38) construction
  line L770 (-26.5, -40.5) -> (-26.5, 40.5)
  point P0 (-23.5, 24.88)
  dimension "d207" = 1
  dimension "d208" = 1
  dimension "d209" = 2.5
  dimension "d210" = 3.7
  constraint horizontal L764
  constraint perpendicular L764 L765
  constraint parallel L764 L766
  constraint parallel L765 L767
  constraint coincident L768 P0
  constraint coincident L769 P0
  measures "d207" distance of L765.end L766.end
  measures "d208" distance of L764.start L766.end
  measures "d209" distance of L767 L770
  measures "d210" distance of L7 L766
extrude "Extrude33" cut sketch "Sketch33" against normal blind 1 contours L764 L765 L766 L767 bodies 1
pattern_linear "R-Pattern11" count 2 spacing 3 along (-1, 0, 0) count 5 spacing 2.63 along (0, -1, 0) of "Extrude33"